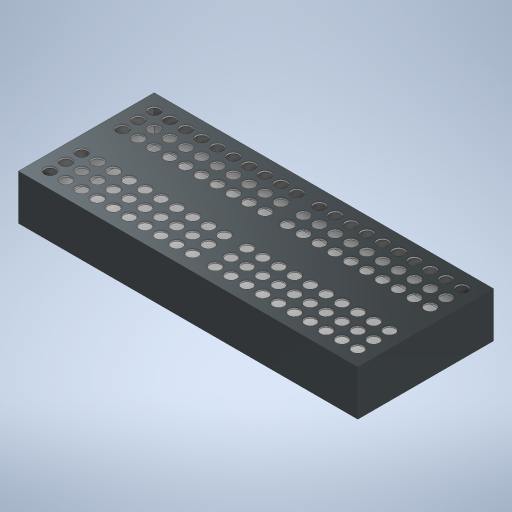
# Autodesk Inventor part: Base
Saved by Autodesk Inventor 2024 (Build 280153000, 153)
## iProperties
Created: 2024-02-01
Part Number: Base
Material: Generic
Document SubType Name: Modeling
Designer: HP
Density: 1 g/cm^3
Appearance: Default
Author: HP
Autodesk Inventor part; units mm, degrees
ref_plane "YZ Plane" through (0, 0, 0) normal (1, 0, 0) x (0, 1, 0)
ref_plane "XZ Plane" through (0, 0, 0) normal (0, 1, 0) x (-1, 0, 0)
ref_plane "XY Plane" through (0, 0, 0) normal (0, 0, 1) x (1, 0, 0)
sketch "Sketch1" plane through (0, 0, 0) normal (1, 0, 0) x (0, 1, 0)
  line L0 (0, 0) -> (100, 0)
  line L1 (100, 0) -> (100, 300)
  line L2 (100, 300) -> (0, 300)
  line L3 (0, 300) -> (0, 0)
  dimension "d0" = 100
  dimension "d1" = 300
  constraints: 8 end point, 2 parallel, 1 horizontal, 1 perpendicular
  measures "d0" distance of L2.end L1.end
  measures "d1" distance of L1.end L0.end
extrude "Extrusion1" add sketch "Sketch1" along normal blind 750
sketch "Sketch2" plane through (0, 100, 300) normal (0, 1, 0) x (1, 0, 0)
  line L0 (3, 3) -> (747, 3)
  line L1 (747, 3) -> (747, 297)
  line L2 (747, 297) -> (3, 297)
  line L3 (3, 297) -> (3, 3)
  point P0 (0, 300)
  dimension "d4" = 744
  dimension "d5" = 294
  constraints: 8 end point, 2 parallel, 1 horizontal, 1 perpendicular
  measures "d4" distance of L2.end L1.end
  measures "d5" distance of L1.end L0.end
extrude "Extrusion2" cut sketch "Sketch2" against normal blind 97
sketch "Sketch3" plane through (0, 100, 300) normal (0, 1, 0) x (1, 0, 0)
  line L0 (0, 0) -> (750, 0)
  line L1 (750, 0) -> (750, 300)
  line L2 (750, 300) -> (0, 300)
  line L3 (0, 300) -> (0, 0)
  dimension "d8" = 750
  dimension "d9" = 300
  constraints: 8 end point, 2 parallel, 1 horizontal, 1 perpendicular
  measures "d8" distance of L2.end L1.end
  measures "d9" distance of L1.end L0.end
extrude "Extrusion3" add sketch "Sketch3" against normal blind 3
sketch "Sketch4" plane through (0, 100, 300) normal (0, 1, 0) x (1, 0, 0)
  circle A0 centre (35, 265) radius 12.5
  circle A1 centre (35, 230) radius 12.5
  circle A2 centre (35, 195) radius 12.5
  circle A3 centre (35, 105) radius 12.5
  circle A4 centre (35, 70) radius 12.5
  circle A5 centre (35, 35) radius 12.5
  circle A6 centre (70, 265) radius 12.5
  circle A7 centre (105, 265) radius 12.5
  circle A8 centre (140, 265) radius 12.5
  circle A9 centre (175, 265) radius 12.5
  circle A10 centre (70, 230) radius 12.5
  circle A11 centre (105, 230) radius 12.5
  circle A12 centre (140, 230) radius 12.5
  circle A13 centre (175, 230) radius 12.5
  circle A14 centre (210, 265) radius 12.5
  circle A15 centre (245, 265) radius 12.5
  circle A16 centre (280, 265) radius 12.5
  circle A17 centre (315, 265) radius 12.5
  circle A18 centre (350, 265) radius 12.5
  circle A19 centre (400, 265) radius 12.5
  circle A20 centre (435, 265) radius 12.5
  circle A21 centre (470, 265) radius 12.5
  circle A22 centre (505, 265) radius 12.5
  circle A23 centre (540, 265) radius 12.5
  circle A24 centre (575, 265) radius 12.5
  circle A25 centre (610, 265) radius 12.5
  circle A26 centre (645, 265) radius 12.5
  circle A27 centre (680, 265) radius 12.5
  circle A28 centre (715, 265) radius 12.5
  circle A29 centre (210, 230) radius 12.5
  circle A30 centre (245, 230) radius 12.5
  circle A31 centre (280, 230) radius 12.5
  circle A32 centre (315, 230) radius 12.5
  circle A33 centre (350, 230) radius 12.5
  circle A34 centre (350, 195) radius 12.5
  circle A35 centre (315, 195) radius 12.5
  circle A36 centre (280, 195) radius 12.5
  circle A37 centre (70, 195) radius 12.5
  circle A38 centre (105, 195) radius 12.5
  circle A39 centre (140, 195) radius 12.5
  circle A40 centre (175, 195) radius 12.5
  circle A41 centre (210, 195) radius 12.5
  circle A42 centre (245, 195) radius 12.5
  circle A43 centre (400, 230) radius 12.5
  circle A44 centre (435, 230) radius 12.5
  circle A45 centre (470, 230) radius 12.5
  circle A46 centre (505, 230) radius 12.5
  circle A47 centre (540, 230) radius 12.5
  circle A48 centre (575, 230) radius 12.5
  circle A49 centre (610, 230) radius 12.5
  circle A50 centre (645, 230) radius 12.5
  circle A51 centre (680, 230) radius 12.5
  circle A52 centre (715, 230) radius 12.5
  circle A53 centre (400, 195) radius 12.5
  circle A54 centre (435, 195) radius 12.5
  circle A55 centre (470, 195) radius 12.5
  circle A56 centre (505, 195) radius 12.5
  circle A57 centre (540, 195) radius 12.5
  circle A58 centre (575, 195) radius 12.5
  circle A59 centre (610, 195) radius 12.5
  circle A60 centre (645, 195) radius 12.5
  circle A61 centre (680, 195) radius 12.5
  circle A62 centre (715, 195) radius 12.5
  circle A63 centre (70, 105) radius 12.5
  circle A64 centre (105, 105) radius 12.5
  circle A65 centre (140, 105) radius 12.5
  circle A66 centre (175, 105) radius 12.5
  circle A67 centre (210, 105) radius 12.5
  circle A68 centre (245, 105) radius 12.5
  circle A69 centre (280, 105) radius 12.5
  circle A70 centre (315, 105) radius 12.5
  circle A71 centre (350, 105) radius 12.5
  circle A72 centre (70, 70) radius 12.5
  circle A73 centre (105, 70) radius 12.5
  circle A74 centre (140, 70) radius 12.5
  circle A75 centre (175, 70) radius 12.5
  circle A76 centre (210, 70) radius 12.5
  circle A77 centre (245, 70) radius 12.5
  circle A78 centre (280, 70) radius 12.5
  circle A79 centre (315, 70) radius 12.5
  circle A80 centre (350, 70) radius 12.5
  circle A81 centre (70, 35) radius 12.5
  circle A82 centre (105, 35) radius 12.5
  circle A83 centre (140, 35) radius 12.5
  circle A84 centre (175, 35) radius 12.5
  circle A85 centre (210, 35) radius 12.5
  circle A86 centre (245, 35) radius 12.5
  circle A87 centre (280, 35) radius 12.5
  circle A88 centre (315, 35) radius 12.5
  circle A89 centre (350, 35) radius 12.5
  circle A90 centre (400, 105) radius 12.5
  circle A91 centre (435, 105) radius 12.5
  circle A92 centre (470, 105) radius 12.5
  circle A93 centre (505, 105) radius 12.5
  circle A94 centre (540, 105) radius 12.5
  circle A95 centre (575, 105) radius 12.5
  circle A96 centre (610, 105) radius 12.5
  circle A97 centre (645, 105) radius 12.5
  circle A98 centre (680, 105) radius 12.5
  circle A99 centre (715, 105) radius 12.5
  circle A100 centre (400, 70) radius 12.5
  circle A101 centre (435, 70) radius 12.5
  circle A102 centre (470, 70) radius 12.5
  circle A103 centre (505, 70) radius 12.5
  circle A104 centre (540, 70) radius 12.5
  circle A105 centre (575, 70) radius 12.5
  circle A106 centre (610, 70) radius 12.5
  circle A107 centre (645, 70) radius 12.5
  circle A108 centre (680, 70) radius 12.5
  circle A109 centre (715, 70) radius 12.5
  circle A110 centre (400, 35) radius 12.5
  circle A111 centre (435, 35) radius 12.5
  circle A112 centre (470, 35) radius 12.5
  circle A113 centre (505, 35) radius 12.5
  circle A114 centre (540, 35) radius 12.5
  circle A115 centre (575, 35) radius 12.5
  circle A116 centre (610, 35) radius 12.5
  circle A117 centre (645, 35) radius 12.5
  circle A118 centre (680, 35) radius 12.5
  circle A119 centre (715, 35) radius 12.5
  point P0 (0, 300)
  dimension "d12" = 25
  dimension "d13" = 25
  dimension "d14" = 25
  dimension "d15" = 25
  dimension "d16" = 25
  dimension "d17" = 25
  constraints: 120 centre point, 25 coincident
  measures "d12" diameter of A0
  measures "d13" diameter of A1
  measures "d14" diameter of A2
  measures "d15" diameter of A3
  measures "d16" diameter of A4
  measures "d17" diameter of A5
extrude "Extrusion4" cut sketch "Sketch4" against normal blind 3
body "Solid1"
